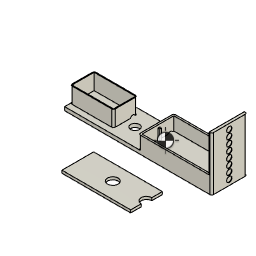
Sppiner drawning v11 (Autodesk Fusion 360 design; units mm, degrees)
Autodesk Fusion 360 part; units mm, degrees
sketch "base principal" plane through (0, 0, 0) normal (0, 0, 1) x (1, 0, 0)
  line L0 (0, 0) -> (107, 0)
  line L1 (107, 0) -> (107, -40)
  line L2 (107, -40) -> (0, -40)
  line L3 (0, -40) -> (0, 0)
  dimension "base_L" = 107
  dimension "base_C" = 40
  constraint horizontal L0
  constraint vertical L1
  constraint horizontal L2
  constraint vertical L3
  constraint coincident L0.start L3.end
  measures "base_L" distance of L0.start L0.end
  measures "base_C" distance of L0.start L2.end
extrude "Extrude5" add sketch "base principal" along normal blind 4 makes body 1
sketch "base LED's" plane through (0, 0, 4) normal (0, 0, 1) x (-1, 0, 0)
  line L0 (0, 40) -> (-107, 40)
  line L1 (-107, 40) -> (-107, 0)
  line L2 (-107, 0) -> (0, 0)
  line L3 (0, 0) -> (0, 40)
  line L4 (-107, 0) -> (-104, 0)
  line L5 (-104, 0) -> (-104, 40)
  line L6 (-104, 40) -> (-107, 40)
  line L7 (-107, 40) -> (-107, 0)
  dimension "baseLED_C" = 3
  dimension "baseLED_L" = 40
  constraint horizontal L4
  constraint vertical L5
  constraint horizontal L6
  constraint vertical L7
  constraint coincident L1.end L2.start
  measures "baseLED_C" distance of L1.end L4.end
  measures "baseLED_L" distance of L1.end L0.end
extrude "Extrude6" add sketch "base LED's" along normal blind 57 contours L0 L1 L2 L4 L5 L6 L7 bodies 1
sketch "base  contrapeso" plane through (0, 0, 4) normal (0, 0, 1) x (-1, 0, 0)
  line L0 (-104, 40) -> (-104, 0)
  line L1 (-104, 0) -> (0, 0)
  line L2 (0, 0) -> (0, 40)
  line L3 (0, 40) -> (-104, 40)
  line L4 (0, 0) -> (60, 0)
  line L5 (60, 0) -> (60, 40)
  line L6 (60, 40) -> (0, 40)
  line L7 (0, 40) -> (0, 0)
  dimension "d27" = 60
  dimension "d28" = 40
  constraint horizontal L4
  constraint vertical L5
  constraint horizontal L6
  constraint vertical L7
  constraint coincident L1.end L2.start
  measures "d27" distance of L1.end L4.end
  measures "d28" distance of L1.end L2.end
extrude "Extrude7" add sketch "base  contrapeso" against normal blind 4 contours L2 L4 L5 L6 L7 bodies 1
sketch "Sketch21" plane through (0, 0, 4) normal (0, 0, 1) x (-1, 0, 0)
  circle A0 centre (0, 20) radius 5
  line L0 (-104, 40) -> (-104, 0)
  line L1 (-104, 0) -> (60, 0)
  line L2 (60, 0) -> (60, 40)
  line L3 (60, 40) -> (-104, 40)
  line L4 (-104, 0) -> (-24, 0)
  line L5 (-24, 0) -> (-24, 2)
  line L6 (-24, 2) -> (-104, 2)
  line L7 (-104, 2) -> (-104, 0)
  line L8 (-104, 40) -> (-24, 40)
  line L9 (-24, 40) -> (-24, 38)
  line L10 (-24, 38) -> (-104, 38)
  line L11 (-104, 38) -> (-104, 40)
  line L12 (-24, 2) -> (-26, 2)
  line L13 (-26, 2) -> (-26, 38)
  line L14 (-26, 38) -> (-24, 38)
  line L15 (-24, 38) -> (-24, 2)
  dimension "d78" = 10
  dimension "d148" = 80
  dimension "d149" = 2
  dimension "d150" = 80
  dimension "d151" = 2
  dimension "d152" = 2
  constraint horizontal L4
  constraint vertical L5
  constraint horizontal L6
  constraint vertical L7
  constraint coincident L0.end L1.start
  constraint horizontal L8
  constraint vertical L9
  constraint horizontal L10
  constraint vertical L11
  constraint coincident L0.start L3.end
  constraint horizontal L12
  constraint vertical L13
  constraint horizontal L14
  constraint vertical L15
  constraint coincident L10 L13.end
  measures "d78" diameter of A0
  measures "d148" distance of L0.end L4.end
  measures "d149" distance of L0.end L6.end
  measures "d150" distance of L0.start L8.end
  measures "d151" distance of L0.start L10.end
  measures "d152" distance of L5.end L12.end
sketch "Sketch12" plane through (107, 0, 0) normal (1, 0, 0) x (0, 1, 0)
  line L0 (-40, 0) -> (0, 0)
  line L1 (0, 0) -> (0, 61)
  line L2 (0, 61) -> (-40, 61)
  line L3 (-40, 61) -> (-40, 0)
sketch "Sketch13" plane through (107, 0, 0) normal (1, 0, 0) x (0, 1, 0)
  circle A0 centre (-20.0088, 55.0247) radius 3
  circle A1 centre (-20.0088, 48.0247) radius 3
  circle A2 centre (-20.0088, 41.0247) radius 3
  circle A3 centre (-20.0088, 34.0247) radius 3
  circle A4 centre (-20.0088, 27.0247) radius 3
  circle A5 centre (-20.0088, 20.0247) radius 3
  circle A6 centre (-20.0088, 13.0247) radius 3
  circle A7 centre (-20.0088, 6.0247) radius 3
  line L0 (-40, 59) -> (-20, 59)
  line L1 (-20, 59) -> (-20, 0)
  dimension "d36" = 6
  dimension "d38" = 6
  dimension "d40" = 6
  dimension "d42" = 6
  dimension "d44" = 6
  dimension "d46" = 6
  dimension "d48" = 6
  dimension "d50" = 6
  dimension "d65" = 7
  dimension "d66" = 7
  dimension "d67" = 7
  dimension "d68" = 7
  dimension "d69" = 7
  dimension "d70" = 7
  dimension "d71" = 7
  dimension "d146" = 20
  constraint horizontal L0
  constraint perpendicular L0 L1
  measures "d36" diameter of A0
  measures "d38" diameter of A1
  measures "d40" diameter of A2
  measures "d42" diameter of A3
  measures "d44" diameter of A4
  measures "d46" diameter of A5
  measures "d48" diameter of A6
  measures "d50" diameter of A7
  measures "d65" distance of A0.centre A1.centre
  measures "d66" distance of A1.centre A2.centre
  measures "d67" distance of A2.centre A3.centre
  measures "d68" distance of A3.centre A4.centre
  measures "d69" distance of A4.centre A5.centre
  measures "d70" distance of A5.centre A6.centre
  measures "d71" distance of A6.centre A7.centre
  measures "d146" distance of L0.start L0.end
extrude "Extrude9" cut sketch "Sketch13" against normal blind 0.5 bodies 1
extrude "Extrude14" cut sketch "Sketch21" against normal blind 4 contours A0 bodies 1
sketch "Sketch29" plane through (0, 0, 0) normal (0, 0, 1) x (1, 0, 0)
  line L0 (0, -67) -> (78, -67)
  line L1 (78, -67) -> (78, -103)
  line L2 (78, -103) -> (0, -103)
  line L3 (0, -103) -> (0, -67)
  circle A0 centre (39.5666, -84.8262) radius 6
  arc A1 (78, -79) -> (78, -91) centre (78, -85) ccw
  dimension "d126" = 78
  dimension "d127" = 36
  dimension "d143" = 12
  constraint horizontal L0
  constraint vertical L1
  constraint horizontal L2
  constraint vertical L3
  constraint coincident L1 A1.start
  constraint coincident L1 A1.end
  constraint midpoint L1 A1.centre
  measures "d126" distance of L0.start L0.end
  measures "d127" distance of L0.start L2.end
  measures "d143" diameter of A0
extrude "Extrude22" add sketch "Sketch29" along normal blind 3 separate body contours L0 L1 L2 L3 A1 makes body 2
extrude "Extrude27" add sketch "Sketch21" along normal blind 15 contours L0 L3 L8 L9 L10 L11 L14 | L0 L1 L4 L5 L6 L7 L12 | L6 L10 L12 L13 L14 L15 bodies 1
sketch "Sketch35" plane through (104, 0, 0) normal (-1, 0, 0) x (0, -1, 0)
  line L0 (38, 19) -> (40, 19)
  line L1 (40, 19) -> (40, 61)
  line L2 (40, 61) -> (0, 61)
  line L3 (0, 61) -> (0, 19)
  line L4 (0, 19) -> (2, 19)
  line L5 (2, 19) -> (2, 4)
  line L6 (2, 4) -> (38, 4)
  line L7 (38, 4) -> (38, 19)
  line L8 (5, 58) -> (35, 58)
  line L9 (35, 58) -> (35, 3)
  line L10 (35, 3) -> (5, 3)
  line L11 (5, 3) -> (5, 58)
  dimension "d155" = 30
  dimension "d156" = 55
  constraint horizontal L8
  constraint vertical L9
  constraint horizontal L10
  constraint vertical L11
  measures "d155" distance of L8.start L8.end
  measures "d156" distance of L8.start L10.end
extrude "Extrude28" cut sketch "Sketch35" against normal blind 1 contours L6 L9 L10 L11 | L6 L8 L9 L11 bodies 1
sketch "Sketch36" plane through (26, 0, 0) normal (1, 0, 0) x (0, 1, 0)
  line L0 (-38, 4) -> (-2, 4)
  line L1 (-2, 4) -> (-2, 19)
  line L2 (-2, 19) -> (-38, 19)
  line L3 (-38, 19) -> (-38, 4)
  arc A0 (-3.1198, 4) -> (-9.4921, 2) centre (-5.9921, 2) ccw
  constraint coincident L0 A0.start
extrude "Extrude29" cut sketch "Sketch36" against normal blind 2 contours L0 A0 bodies 1
sketch "Sketch37" plane through (0, 0, 4) normal (0, 0, 1) x (-1, 0, 0)
  circle A0 centre (0, 20) radius 5
  line L0 (-26, 38) -> (-104, 38)
  line L1 (-104, 38) -> (-104, 35)
  line L2 (-104, 2) -> (-26, 2)
  line L3 (-26, 2) -> (-26, 3.1198)
  line L4 (-26, 3.1198) -> (-24, 3.1198)
  line L5 (-24, 3.1198) -> (-24, 0)
  line L6 (-24, 0) -> (60, 0)
  line L7 (60, 0) -> (60, 40)
  line L8 (60, 40) -> (-24, 40)
  line L9 (-24, 40) -> (-24, 8.8644)
  line L10 (-24, 8.8644) -> (-26, 8.8644)
  line L11 (-26, 8.8644) -> (-26, 38)
  line L12 (-26, 19.9626) -> (-28, 19.9626)
  line L13 (-28, 19.9626) -> (-28, 17.9626)
  line L14 (-28, 17.9626) -> (-26, 17.9626)
  line L15 (-26, 17.9626) -> (-26, 19.9626)
  line L16 (-104, 35) -> (-102, 35)
  line L17 (-102, 35) -> (-102, 37)
  line L18 (-102, 37) -> (-104, 37)
  line L19 (-104, 37) -> (-104, 35)
  line L20 (-104, 38) -> (-102, 38)
  line L21 (-102, 38) -> (-102, 36)
  line L22 (-102, 36) -> (-104, 36)
  line L23 (-104, 36) -> (-104, 38)
  line L24 (-104, 35) -> (-104, 5)
  line L25 (-104, 5) -> (-104, 2)
  dimension "d161" = 2
  dimension "d162" = 2
  dimension "d163" = 2
  dimension "d164" = 2
  dimension "d165" = 2
  dimension "d166" = 2
  constraint horizontal L12
  constraint vertical L13
  constraint horizontal L14
  constraint vertical L15
  constraint coincident L11 L12.start
  constraint horizontal L16
  constraint vertical L17
  constraint horizontal L18
  constraint vertical L19
  constraint coincident L1.end L16.start
  constraint horizontal L20
  constraint vertical L21
  constraint horizontal L22
  constraint vertical L23
  constraint coincident L0.end L1.start
  measures "d161" distance of L12.start L12.end
  measures "d162" distance of L12.start L14.end
  measures "d163" distance of L1.end L16.end
  measures "d164" distance of L1.end L18.end
  measures "d165" distance of L0.end L20.end
  measures "d166" distance of L0.end L22.end
extrude "Extrude30" add sketch "Sketch37" along normal blind 12 contours L0 L1 L18 L20 L21 L23 | L11 L12 L13 L14 L15 | L1 L17 L18 L19 L21 L22 L23 | L1 L16 L17 L19 L22 bodies 1
sketch "Sketch38" plane through (0, 0, 4) normal (0, 0, 1) x (-1, 0, 0)
  line L0 (-104, 2) -> (-26, 2)
  line L1 (-26, 2) -> (-26, 3.1198)
  line L2 (-26, 3.1198) -> (-24, 3.1198)
  line L3 (-24, 3.1198) -> (-24, 0)
  line L4 (-24, 0) -> (60, 0)
  line L5 (60, 0) -> (60, 40)
  line L6 (60, 40) -> (-24, 40)
  line L7 (-24, 40) -> (-24, 8.8644)
  line L8 (-24, 8.8644) -> (-26, 8.8644)
  line L9 (-26, 8.8644) -> (-26, 17.9626)
  line L10 (-26, 17.9626) -> (-28, 17.9626)
  line L11 (-28, 17.9626) -> (-28, 19.9626)
  line L12 (-28, 19.9626) -> (-26, 19.9626)
  line L13 (-26, 19.9626) -> (-26, 38)
  line L14 (-26, 38) -> (-102, 38)
  line L15 (-102, 38) -> (-102, 35)
  line L16 (-104, 5) -> (-104, 2)
  circle A0 centre (0, 20) radius 5
  line L17 (60, 0) -> (60, 1.6)
  line L18 (60, 1.6) -> (11, 1.6)
  line L19 (11, 1.6) -> (11, 38.6)
  line L20 (11, 38.6) -> (60, 38.6)
  line L21 (60, 38.6) -> (60, 1.6)
  line L22 (-102, 35) -> (-104, 35)
  line L23 (-104, 35) -> (-104, 5)
  dimension "d176" = 1.6
  dimension "d177" = 49
  dimension "d178" = 37
  constraint coincident L4.end L5.start
  constraint vertical L17
  constraint horizontal L18
  constraint vertical L19
  constraint horizontal L20
  constraint vertical L21
  measures "d176" distance of L4.end L17.end
  measures "d177" distance of L17.end L18.end
  measures "d178" distance of L17.end L20.end
sketch "Sketch40" plane through (0, 0, 4) normal (0, 0, 1) x (-1, 0, 0)
  line L0 (-28, 19.9626) -> (-26, 19.9626)
  line L1 (-26, 19.9626) -> (-26, 38)
  line L2 (-26, 38) -> (-102, 38)
  line L3 (-102, 38) -> (-102, 35)
  line L4 (-102, 35) -> (-104, 35)
  line L5 (-104, 35) -> (-104, 5)
  line L6 (-104, 5) -> (-104, 2)
  line L7 (-104, 2) -> (-26, 2)
  line L8 (-26, 2) -> (-26, 3.1198)
  line L9 (-26, 3.1198) -> (-24, 3.1198)
  line L10 (-24, 3.1198) -> (-24, 0)
  line L11 (-24, 0) -> (60, 0)
  line L12 (60, 0) -> (60, 40)
  line L13 (60, 40) -> (-24, 40)
  line L14 (-24, 40) -> (-24, 8.8644)
  line L15 (-24, 8.8644) -> (-26, 8.8644)
  line L16 (-26, 8.8644) -> (-26, 17.9626)
  line L17 (-26, 17.9626) -> (-28, 17.9626)
  line L18 (-28, 17.9626) -> (-28, 19.9626)
  circle A0 centre (0, 20) radius 5
  line L19 (60, 0) -> (60, 6.5)
  line L20 (60, 6.5) -> (11, 6.5)
  line L21 (11, 6.5) -> (11, 33.5)
  line L22 (11, 33.5) -> (60, 33.5)
  line L23 (60, 33.5) -> (60, 6.5)
  dimension "d187" = 6.5
  dimension "d188" = 49
  dimension "d189" = 27
  constraint coincident L11.end L12.start
  constraint perpendicular L11 L19
  constraint horizontal L20
  constraint vertical L21
  constraint horizontal L22
  constraint vertical L23
  measures "d187" distance of L11.end L19.end
  measures "d188" distance of L19.end L20.end
  measures "d189" distance of L19.end L22.end
extrude "Extrude33" add sketch "Sketch40" along normal blind 18 thin wall 1 inside contours L12 L20 L21 L22 L23 bodies 1
fillet "Fillet3" radius 2 4 edges at (107, 0, 30.5) (107, -40, 30.5) (24, -40, 11.5) (24, 0, 11.5) on bodies 1
fillet "Fillet3" radius 2 4 edges at (-11, -6.5, 13) (-11, -33.5, 13) (-60, -6.5, 13) (-60, -33.5, 13) on bodies 1
sketch "Sketch42" plane through (-11, 0, 0) normal (1, 0, 0) x (0, 1, 0)
  line L0 (-31.5, 22) -> (-31.5, 4)
  line L1 (-31.5, 4) -> (-8.5, 4)
  line L2 (-8.5, 4) -> (-8.5, 22)
  line L3 (-8.5, 22) -> (-31.5, 22)
  arc A0 (-8.5, 4) -> (-14.245, 4) centre (-11.3725, 3.1275) ccw
  constraint coincident L1.end L2.start
extrude "Extrude35" cut sketch "Sketch42" against normal blind 2 contours L1 A0 bodies 1
equation "h_base = 4 mm"
equation "H_LED = 57 mm"
equation "h_suporte = 10 mm"
